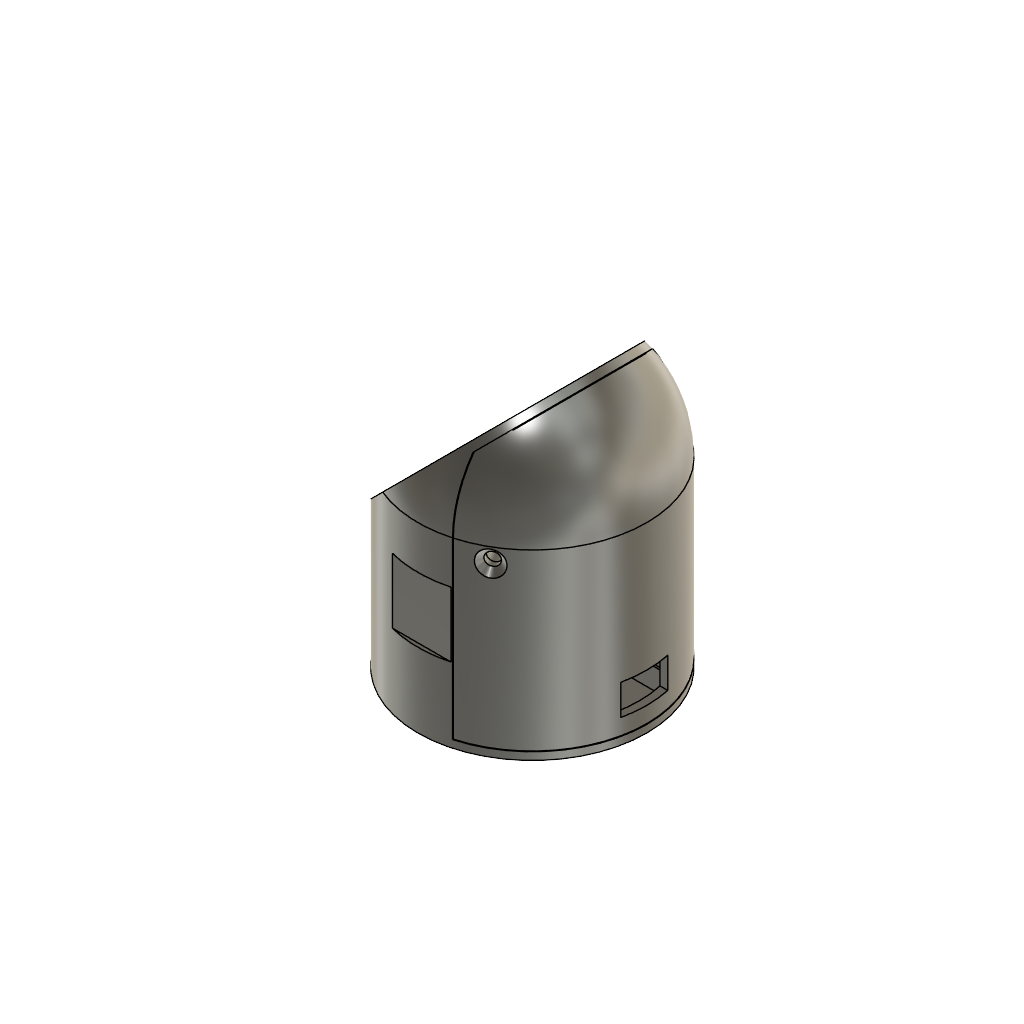
claude_toy (Autodesk Fusion 360 archive; units mm, degrees)
design "claude_bot"
Autodesk Fusion 360 part; units mm, degrees
sketch "Esquisse1" plane through (0, 0, 0) normal (0, 1, 0) x (1, 0, 0)
  line L0 (0, 0) -> (30, 0)
  line L1 (30, 0) -> (30, -47.81)
  arc A0 (0, -77.81) -> (30, -47.81) centre (0, -47.81) ccw
  arc A1 (0, -75.81) -> (28, -47.81) centre (0, -47.81) ccw
  line L2 (28, -2) -> (28, -47.81)
  line L3 (0, -2) -> (28, -2)
  line L4 (0, -77.81) -> (0, -75.81)
  line L5 (0, -2) -> (0, 0)
  line L6 (-0.0898, 1.012) -> (-0.0898, -78.988) construction
  dimension "d3" = 2
  dimension "d17" = 30
  constraint coincident L0.start L5.end
  constraint horizontal L0
  constraint perpendicular L0 L1
  constraint tangent L1 A0
  constraint perpendicular A1 L4
  constraint perpendicular L0 L5
  constraint perpendicular L3 L6
  constraint parallel L4 L6
  constraint coincident L0.start L4
  measures "d17" distance of L0.start L0.end
revolve "Révolution1" add sketch "Esquisse1" angle 360 about axis through (0, 0, 1.75) along (0, 0, 1) makes body 1
ref_plane "Plan de construction4" through (0, 12.125, 0) normal (-0.707107, 0, 0.707107) x (0, 1, 0)
ref_plane "Plan de construction5" through (-28.2843, 12.125, 28.2843) normal (-0.707107, 0, 0.707107) x (0, 1, 0)
split "Scinder1" by plane through (-28.2843, 12.125, 28.2843) normal (-0.707107, 0, 0.707107) bodies 1 makes body 2 at (-10.3059, -28.0164, 50.7878)
sketch "Esquisse3" plane through (-28.2843, 0, 28.2843) normal (-0.707107, 0, 0.707107) x (0, -1, 0)
  ellipse E0 centre (0, 40) end of major axis (0, 82.4264) minor radius 30 (-28.693, 27.6136) -> (28.693, 27.6136) ccw
  arc A0 (28.693, 27.6136) -> (-28.693, 27.6136) centre (0, 33.8068) ccw
  ellipse E1 centre (0, 40) end of major axis (0, 79.598) minor radius 28 (-26.5949, 27.6136) -> (26.5949, 27.6136) ccw
  arc A1 (26.5949, 27.6136) -> (-26.5949, 27.6136) centre (0, 33.8068) ccw
extrude "Extrusion1" add sketch "Esquisse3" along normal blind 2 separate body contours E1 A1 makes body 3
sketch "Esquisse4" plane through (-29.6985, 0, 29.6985) normal (-0.707107, 0, 0.707107) x (0, -1, 0)
  arc A0 (26.5949, 27.6136) -> (-26.5949, 27.6136) centre (0, 33.8068) ccw
  ellipse E0 centre (0, 40) end of major axis (0, 79.598) minor radius 28 (-26.5949, 27.6136) -> (26.5949, 27.6136) ccw
  arc A1 (7.706, 19.3175) -> (-9.294, 19.3175) centre (-0.794, 34.9574) ccw
  line L0 (-9.294, 19.3175) -> (-7.394, 14.6576)
  line L1 (-7.394, 14.6576) -> (-7.394, 14.157)
  line L2 (-7.394, 14.157) -> (5.806, 14.157)
  line L3 (5.806, 14.157) -> (5.806, 14.6576)
  line L4 (5.806, 14.6576) -> (7.706, 19.3175)
  line L5 (-9.4523, 19.176) -> (-7.594, 14.6184)
  line L6 (-7.594, 14.6184) -> (-7.594, 13.957)
  line L7 (-7.594, 13.957) -> (6.006, 13.957)
  line L8 (6.006, 13.957) -> (6.006, 14.6184)
  line L9 (6.006, 14.6184) -> (7.8643, 19.176)
  arc A2 (7.8643, 19.176) -> (-9.4523, 19.176) centre (-0.794, 34.9574) ccw
  dimension "d18" = 0.2
extrude "Decoupe ecran" cut sketch "Esquisse4" against normal blind 3 contours A1 L0 L1 L2 L3 L4 | L5 L6 L7 L8 L9 A2 bodies 3
ref_plane "Plan de construction6" through (0, 26, 0) normal (0, 1, 0) x (0, 0, 1)
sketch "Esquisse8" plane through (0, 26, 0) normal (0, 1, 0) x (1, 0, 0)
  line L0 (-7.5, -18.5) -> (7.5, -18.5)
  line L1 (7.5, -18.5) -> (7.5, -37.5)
  line L2 (7.5, -37.5) -> (-7.5, -37.5)
  line L3 (-7.5, -37.5) -> (-7.5, -18.5)
extrude "Bossage capteur droite" add sketch "Esquisse8" along normal blind 3 bodies 1
ref_plane "Plan de construction7" through (0, 29, 0) normal (0, 1, 0) x (0, 0, 1)
sketch "Esquisse9" plane through (0, 29, 0) normal (0, 1, 0) x (1, 0, 0)
  line L0 (-9, -19.5) -> (9, -19.5)
  line L1 (9, -19.5) -> (9, -36.5)
  line L2 (9, -36.5) -> (-9, -36.5)
  line L3 (-9, -36.5) -> (-9, -19.5)
extrude "Meplat capteur droite" cut sketch "Esquisse9" along normal blind 2 bodies 1
ref_plane "Plan de construction8" through (0, 25.5, 0) normal (0, 1, 0) x (0, 0, 1)
sketch "Esquisse10" plane through (0, 25.5, 0) normal (0, 1, 0) x (1, 0, 0)
  line L0 (-5.53, -20.6) -> (5.53, -20.6)
  line L1 (5.53, -20.6) -> (5.53, -35.4)
  line L2 (5.53, -35.4) -> (-5.53, -35.4)
  line L3 (-5.53, -35.4) -> (-5.53, -20.6)
extrude "Logement capteur droite" cut sketch "Esquisse10" along normal blind 3 bodies 1
ref_plane "Plan de construction9" through (0, -26, 0) normal (0, 1, 0) x (0, 0, 1)
sketch "Esquisse11" plane through (0, -26, 0) normal (0, 1, 0) x (1, 0, 0)
  line L0 (-7.5, -18.5) -> (7.5, -18.5)
  line L1 (7.5, -18.5) -> (7.5, -37.5)
  line L2 (7.5, -37.5) -> (-7.5, -37.5)
  line L3 (-7.5, -37.5) -> (-7.5, -18.5)
extrude "Bossage capteur gauche" add sketch "Esquisse11" against normal blind 3 bodies 1
ref_plane "Plan de construction10" through (0, -29, 0) normal (0, 1, 0) x (0, 0, 1)
sketch "Esquisse12" plane through (0, -29, 0) normal (0, 1, 0) x (1, 0, 0)
  line L0 (-9, -19.5) -> (9, -19.5)
  line L1 (9, -19.5) -> (9, -36.5)
  line L2 (9, -36.5) -> (-9, -36.5)
  line L3 (-9, -36.5) -> (-9, -19.5)
extrude "Meplat capteur gauche" cut sketch "Esquisse12" against normal blind 2 bodies 1
ref_plane "Plan de construction11" through (0, -25.5, 0) normal (0, 1, 0) x (0, 0, 1)
sketch "Esquisse13" plane through (0, -25.5, 0) normal (0, 1, 0) x (1, 0, 0)
  line L0 (-5.53, -20.6) -> (5.53, -20.6)
  line L1 (5.53, -20.6) -> (5.53, -35.4)
  line L2 (5.53, -35.4) -> (-5.53, -35.4)
  line L3 (-5.53, -35.4) -> (-5.53, -20.6)
extrude "Logement capteur gauche" cut sketch "Esquisse13" against normal blind 3 bodies 1
ref_plane "Plan de construction12" through (0, 0, 1) normal (0, 0, 1) x (1, 0, 0)
sketch "Esquisse14" plane through (0, 0, 1) normal (0, 0, 1) x (1, 0, 0)
  line L0 (2.55, 9.15) -> (25.4, 9.15)
  line L1 (25.4, 9.15) -> (25.4, 10.65)
  line L2 (25.4, 10.65) -> (2.55, 10.65)
  line L3 (2.55, 10.65) -> (2.55, 9.15)
  line L4 (2.55, -10.65) -> (25.4, -10.65)
  line L5 (25.4, -10.65) -> (25.4, -9.15)
  line L6 (25.4, -9.15) -> (2.55, -9.15)
  line L7 (2.55, -9.15) -> (2.55, -10.65)
  line L8 (1.05, -10.65) -> (2.55, -10.65)
  line L9 (2.55, -10.65) -> (2.55, 10.65)
  line L10 (2.55, 10.65) -> (1.05, 10.65)
  line L11 (1.05, 10.65) -> (1.05, -10.65)
extrude "Berceau ESP parois" add sketch "Esquisse14" along normal blind 9.1 bodies 1
ref_plane "Plan de construction13" through (0, 0, 1) normal (0, 0, 1) x (1, 0, 0)
sketch "Esquisse15" plane through (0, 0, 1) normal (0, 0, 1) x (1, 0, 0)
  line L0 (2.7, 8.6) -> (25.4, 8.6)
  line L1 (25.4, 8.6) -> (25.4, 9.15)
  line L2 (25.4, 9.15) -> (2.7, 9.15)
  line L3 (2.7, 9.15) -> (2.7, 8.6)
  line L4 (2.7, -9.15) -> (25.4, -9.15)
  line L5 (25.4, -9.15) -> (25.4, -8.6)
  line L6 (25.4, -8.6) -> (2.7, -8.6)
  line L7 (2.7, -8.6) -> (2.7, -9.15)
extrude "Berceau ESP appuis" add sketch "Esquisse15" along normal blind 6.5 bodies 1
ref_plane "Plan de construction14" through (0, 0, 9.21) normal (0, 0, 1) x (1, 0, 0)
sketch "Esquisse16" plane through (0, 0, 9.21) normal (0, 0, 1) x (1, 0, 0)
  line L0 (12.45, 8.6) -> (16.45, 8.6)
  line L1 (16.45, 8.6) -> (16.45, 9.15)
  line L2 (16.45, 9.15) -> (12.45, 9.15)
  line L3 (12.45, 9.15) -> (12.45, 8.6)
  line L4 (12.45, -9.15) -> (16.45, -9.15)
  line L5 (16.45, -9.15) -> (16.45, -8.6)
  line L6 (16.45, -8.6) -> (12.45, -8.6)
  line L7 (12.45, -8.6) -> (12.45, -9.15)
extrude "Clips ESP" add sketch "Esquisse16" along normal blind 0.4 bodies 1
ref_plane "Plan de construction15" through (27, 0, 0) normal (1, 0, 0) x (0, 1, 0)
sketch "Esquisse18" plane through (0, 0, 9.21) normal (0, 0, 1) x (1, 0, 0)
  line L0 (12.45, 8.6) -> (16.45, 8.6)
  line L1 (16.45, 8.6) -> (16.45, 8.85)
  line L2 (16.45, 8.85) -> (12.45, 8.85)
  line L3 (12.45, 8.85) -> (12.45, 8.6)
  line L4 (12.45, -8.85) -> (16.45, -8.85)
  line L5 (16.45, -8.85) -> (16.45, -8.6)
  line L6 (16.45, -8.6) -> (12.45, -8.6)
  line L7 (12.45, -8.6) -> (12.45, -8.85)
extrude "Clips ESP extension" add sketch "Esquisse18" along normal blind 0.4 bodies 1
sketch "Esquisse19" plane through (27, 0, 0) normal (1, 0, 0) x (0, 0, -1)
  line L0 (-6.31, -6.15) -> (-14.31, -6.15)
  line L1 (-14.31, -6.15) -> (-14.31, 6.15)
  line L2 (-14.31, 6.15) -> (-6.31, 6.15)
  line L3 (-6.31, 6.15) -> (-6.31, -6.15)
extrude "Passage USB-C" cut sketch "Esquisse19" along normal blind 4 bodies 1
ref_plane "Plan de construction16" through (0, 28.5, 0) normal (0, 1, 0) x (0, 0, 1)
ref_plane "Plan de construction17" through (0, -28.5, 0) normal (0, 1, 0) x (0, 0, 1)
ref_plane "Plan de construction18" through (0, 0, 2) normal (0, 0, 1) x (1, 0, 0)
ref_plane "Plan de construction19" through (0, 0, 2.15) normal (0, 0, 1) x (1, 0, 0)
sketch "Esquisse22" plane through (0, 0, 2) normal (0, 0, 1) x (1, 0, 0)
  line L0 (8, -31) -> (31, -31)
  line L1 (31, -31) -> (31, 31)
  line L2 (31, 31) -> (8, 31)
  line L3 (8, 31) -> (8, -31)
extrude "Outil coupe principal" add sketch "Esquisse22" along normal blind 78 separate body makes body 4
sketch "Esquisse23" plane through (0, 0, 2) normal (0, 0, 1) x (1, 0, 0)
  line L0 (8, -11) -> (25.5, -11)
  line L1 (25.5, -11) -> (25.5, 11)
  line L2 (25.5, 11) -> (8, 11)
  line L3 (8, 11) -> (8, -11)
extrude "Outil reserve berceau" cut sketch "Esquisse23" along normal blind 9 bodies 4
sketch "Esquisse24" plane through (0, 0, 2.15) normal (0, 0, 1) x (1, 0, 0)
  line L0 (8.15, -31) -> (31, -31)
  line L1 (31, -31) -> (31, 31)
  line L2 (31, 31) -> (8.15, 31)
  line L3 (8.15, 31) -> (8.15, -31)
extrude "Outil coupe trappe" add sketch "Esquisse24" along normal blind 77.85 separate body makes body 5
sketch "Esquisse25" plane through (0, 0, 2.15) normal (0, 0, 1) x (1, 0, 0)
  line L0 (8, -11.15) -> (25.65, -11.15)
  line L1 (25.65, -11.15) -> (25.65, 11.15)
  line L2 (25.65, 11.15) -> (8, 11.15)
  line L3 (8, 11.15) -> (8, -11.15)
extrude "Outil reserve berceau jeu" cut sketch "Esquisse25" along normal blind 9 bodies 5
sketch "Esquisse26" plane through (0, 0, 0) normal (0, 1, 0) x (1, 0, 0)
  line L0 (5, -61.3564) -> (40, -96.3564)
  line L1 (40, -96.3564) -> (5, -96.3564)
  line L2 (5, -96.3564) -> (5, -61.3564)
extrude "Outil jeu facade" cut sketch "Esquisse26" along normal mid plane 35 bodies 5
sketch "Esquisse37" plane through (0, 0, 0) normal (0, 1, 0) x (1, 0, 0)
  line L0 (28, -2) -> (29, -2)
  line L1 (29, -2) -> (29, -47.81)
  arc A0 (0, -76.81) -> (29, -47.81) centre (0, -47.81) ccw
  line L2 (0, -76.81) -> (0, -75.81)
  arc A1 (0, -75.81) -> (28, -47.81) centre (0, -47.81) ccw
  line L3 (28, -47.81) -> (28, -2)
revolve "Outil levre principal" add sketch "Esquisse37" angle 360 about axis through (0, 0, 1.75) along (0, 0, 1) separate body makes body 6
ref_plane "Plan de construction25" through (0, 0, 1) normal (0, 0, 1) x (1, 0, 0)
sketch "Esquisse38" plane through (0, 0, 1) normal (0, 0, 1) x (1, 0, 0)
  line L0 (8, -32) -> (11, -32)
  line L1 (11, -32) -> (11, 32)
  line L2 (11, 32) -> (8, 32)
  line L3 (8, 32) -> (8, -32)
extrude "Boite levre principal" add sketch "Esquisse38" along normal blind 80 separate body makes body 7
combine "Levre principal limite" operation intersect target body 6 tool bodies 7
sketch "Esquisse39" plane through (0, 0, 0) normal (0, 1, 0) x (1, 0, 0)
  line L0 (27.85, -1.9) -> (29.15, -1.9)
  line L1 (29.15, -1.9) -> (29.15, -47.81)
  arc A0 (0, -76.96) -> (29.15, -47.81) centre (0, -47.81) ccw
  line L2 (0, -76.96) -> (0, -75.66)
  arc A1 (0, -75.66) -> (27.85, -47.81) centre (0, -47.81) ccw
  line L3 (27.85, -47.81) -> (27.85, -1.9)
revolve "Outil levre trappe" add sketch "Esquisse39" angle 360 about axis through (0, 0, 1.75) along (0, 0, 1) separate body makes body 8
ref_plane "Plan de construction26" through (0, 0, 1) normal (0, 0, 1) x (1, 0, 0)
sketch "Esquisse40" plane through (0, 0, 1) normal (0, 0, 1) x (1, 0, 0)
  line L0 (7, -32) -> (11.15, -32)
  line L1 (11.15, -32) -> (11.15, 32)
  line L2 (11.15, 32) -> (7, 32)
  line L3 (7, 32) -> (7, -32)
extrude "Boite levre trappe" add sketch "Esquisse40" along normal blind 80 separate body makes body 9
combine "Levre trappe limite" operation intersect target body 8 tool bodies 9
combine "Outil principal moins levre" operation cut target body 4 tool bodies 6
combine "Outil trappe moins rainure" operation cut target body 5 tool bodies 8
copy_body "CopierCollerCorps1" bodies 1 makes body 10
combine "Creation trappe" operation intersect target body 10 tool bodies 5
combine "Separation trappe" operation cut target body 1 tool bodies 4
ref_plane "Plan de construction20" through (0, 0, 39) normal (0, 0, 1) x (1, 0, 0)
ref_plane "Plan de construction21" through (0, 0, 40) normal (0, 0, 1) x (1, 0, 0)
sketch "Esquisse27" plane through (0, 0, 39) normal (0, 0, 1) x (1, 0, 0)
  arc A0 (13.6271, 16.2401) -> (1.8477, 21.1193) centre (0, 0) ccw
  arc A1 (17.1624, 20.4534) -> (2.3271, 26.5984) centre (0, 0) ccw
  line L0 (13.6271, 16.2401) -> (17.1624, 20.4534)
  line L1 (1.8477, 21.1193) -> (2.3271, 26.5984)
extrude "Patte vis gauche" add sketch "Esquisse27" along normal blind 10 bodies 1 makes body 11
sketch "Esquisse28" plane through (0, 0, 39) normal (0, 0, 1) x (1, 0, 0)
  arc A0 (6.8587, 25.597) -> (2.3096, 26.3992) centre (0, 0) ccw
  arc A1 (7.6352, 28.4948) -> (2.5711, 29.3877) centre (0, 0) ccw
  line L0 (6.8587, 25.597) -> (7.6352, 28.4948)
  line L1 (2.3096, 26.3992) -> (2.5711, 29.3877)
extrude "Attache patte gauche" add sketch "Esquisse28" along normal blind 10 bodies 1
sketch "Esquisse30" plane through (0, 0, 39) normal (0, 0, 1) x (1, 0, 0)
  arc A0 (1.8477, -21.1193) -> (13.6271, -16.2401) centre (0, 0) ccw
  arc A1 (2.3271, -26.5984) -> (17.1624, -20.4534) centre (0, 0) ccw
  line L0 (13.6271, -16.2401) -> (17.1624, -20.4534)
  line L1 (1.8477, -21.1193) -> (2.3271, -26.5984)
extrude "Patte vis droite" add sketch "Esquisse30" along normal blind 10 bodies 1 makes body 12
sketch "Esquisse31" plane through (0, 0, 39) normal (0, 0, 1) x (1, 0, 0)
  arc A0 (2.3096, -26.3992) -> (6.8587, -25.597) centre (0, 0) ccw
  arc A1 (2.5711, -29.3877) -> (7.6352, -28.4948) centre (0, 0) ccw
  line L0 (6.8587, -25.597) -> (7.6352, -28.4948)
  line L1 (2.3096, -26.3992) -> (2.5711, -29.3877)
extrude "Attache patte droite" add sketch "Esquisse31" along normal blind 10 bodies 1
combine "Fusion pattes vis" operation add target body 1 tool bodies 11 12
sketch "Esquisse41" plane through (0, 0, 40) normal (0, 0, 1) x (1, 0, 0)
  arc A0 (16.1587, 21.4434) -> (11.3473, 24.3344) centre (0, 0) ccw
  arc A1 (17.6332, 23.4) -> (12.3827, 26.5548) centre (0, 0) ccw
  line L0 (16.1587, 21.4434) -> (17.6332, 23.4)
  line L1 (11.3473, 24.3344) -> (12.3827, 26.5548)
extrude "Bossage vis trappe gauche" add sketch "Esquisse41" along normal blind 8 bodies 10
sketch "Esquisse42" plane through (0, 0, 40) normal (0, 0, 1) x (1, 0, 0)
  arc A0 (11.3473, -24.3344) -> (16.1587, -21.4434) centre (0, 0) ccw
  arc A1 (12.3827, -26.5548) -> (17.6332, -23.4) centre (0, 0) ccw
  line L0 (16.1587, -21.4434) -> (17.6332, -23.4)
  line L1 (11.3473, -24.3344) -> (12.3827, -26.5548)
extrude "Bossage vis trappe droite" add sketch "Esquisse42" along normal blind 8 bodies 10
ref_plane "Plan de construction22" through (0, 0, 12.125) normal (-0.866025, 0.5, 0) x (0, 0, 1)
sketch "Esquisse33" plane through (0, 0, 0) normal (-0.866025, 0.5, 0) x (0, 0, 1)
  line L0 (44, 15) -> (44, 33) construction
  line L1 (44, 26.4) -> (45.7, 26.4)
  line L2 (45.7, 26.4) -> (45.7, 28.4)
  line L3 (45.7, 28.4) -> (47.3, 30)
  line L4 (47.3, 30) -> (47.3, 31.5)
  line L5 (47.3, 31.5) -> (44, 31.5)
  line L6 (44, 31.5) -> (44, 26.4)
revolve "Percage fraise trappe gauche" cut sketch "Esquisse33" angle 360 about axis through (7.5, 12.9904, 44) along (0.5, 0.866025, 0) bodies 10
sketch "Esquisse34" plane through (0, 0, 0) normal (-0.866025, 0.5, 0) x (0, 0, 1)
  line L0 (44, 15) -> (44, 33) construction
  line L1 (44, 27) -> (46, 27)
  line L2 (46, 27) -> (46, 22.2)
  line L3 (46, 22.2) -> (45.4, 22.2)
  line L4 (45.4, 22.2) -> (45.4, 20.5)
  line L5 (45.4, 20.5) -> (44, 20.5)
  line L6 (44, 20.5) -> (44, 27)
revolve "Logement insert gauche" cut sketch "Esquisse34" angle 360 about axis through (7.5, 12.9904, 44) along (0.5, 0.866025, 0) bodies 1
ref_plane "Plan de construction24" through (0, 0, 12.125) normal (0.866025, 0.5, 0) x (0, 0, 1)
sketch "Esquisse35" plane through (0, 0, 0) normal (0.866025, 0.5, 0) x (0, 0, 1)
  line L0 (44, 15) -> (44, 33) construction
  line L1 (44, 26.4) -> (45.7, 26.4)
  line L2 (45.7, 26.4) -> (45.7, 28.4)
  line L3 (45.7, 28.4) -> (47.3, 30)
  line L4 (47.3, 30) -> (47.3, 31.5)
  line L5 (47.3, 31.5) -> (44, 31.5)
  line L6 (44, 31.5) -> (44, 26.4)
revolve "Percage fraise trappe droite" cut sketch "Esquisse35" angle 360 about axis through (7.5, -12.9904, 44) along (0.5, -0.866025, 0) bodies 10
sketch "Esquisse36" plane through (0, 0, 0) normal (0.866025, 0.5, 0) x (0, 0, 1)
  line L0 (44, 15) -> (44, 33) construction
  line L1 (44, 27) -> (46, 27)
  line L2 (46, 27) -> (46, 22.2)
  line L3 (46, 22.2) -> (45.4, 22.2)
  line L4 (45.4, 22.2) -> (45.4, 20.5)
  line L5 (45.4, 20.5) -> (44, 20.5)
  line L6 (44, 20.5) -> (44, 27)
revolve "Logement insert droite" cut sketch "Esquisse36" angle 360 about axis through (7.5, -12.9904, 44) along (0.5, -0.866025, 0) bodies 1
combine "Fusion corps + facade" operation add target body 1 tool bodies 3
split "Decoupe anneau facade" by plane through (-29.6985, 0, 29.6985) normal (-0.707107, 0, 0.707107) bodies 2 makes body 13 at (-29.7433, 0, 51.7258)
delete_body "RemoveBody2" bodies 13
combine "Fusion anneau facade" operation add target body 1 tool bodies 2
ref_plane "Plan de construction27" through (-28.2843, 12.125, 28.2843) normal (-0.707107, 0, 0.707107) x (0, 1, 0)
sketch "Esquisse43" plane through (-28.2843, 0, 28.2843) normal (-0.707107, 0, 0.707107) x (0, 1, 0)
  line L0 (-10.936, -9.422) -> (-10.936, -19.2327)
  arc A0 (-10.936, -19.2327) -> (12.524, -19.2327) centre (0.794, -34.622) ccw
  line L1 (12.524, -19.2327) -> (12.524, -9.422)
  arc A1 (12.524, -9.422) -> (10.974, -7.872) centre (10.974, -9.422) ccw
  line L2 (10.974, -7.872) -> (-9.386, -7.872)
  arc A2 (-9.386, -7.872) -> (-10.936, -9.422) centre (-9.386, -9.422) ccw
extrude "Lamage ecran" cut sketch "Esquisse43" along normal blind 0.9 bodies 1
ref_plane "Plan de construction28" through (-28.9207, 12.125, 28.9207) normal (-0.707107, 0, 0.707107) x (0, 1, 0)
sketch "Esquisse44" plane through (-28.9207, 0, 28.9207) normal (-0.707107, 0, 0.707107) x (0, 1, 0)
  circle A0 centre (-8.636, -12.952) radius 2.25
  circle A1 centre (-8.636, -12.952) radius 0.9
  circle A2 centre (10.224, -12.952) radius 2.25
  circle A3 centre (10.224, -12.952) radius 0.9
extrude "Epaulements plots" add sketch "Esquisse44" against normal blind 0.5 contours A0 | A1 | A2 | A3 bodies 1
extrude "Pions scellage" add sketch "Esquisse44" against normal blind 3.6 contours A1 | A3 bodies 1
sketch "Esquisse45" plane through (-28.9207, 0, 28.9207) normal (-0.707107, 0, 0.707107) x (0, 1, 0)
  line L0 (-8, -7.95) -> (9.6, -7.95)
  line L1 (9.6, -7.95) -> (9.6, -11.15)
  line L2 (9.6, -11.15) -> (-8, -11.15)
  line L3 (-8, -11.15) -> (-8, -7.95)
  line L4 (-5.21, -12.5) -> (6.79, -12.5)
  line L5 (6.79, -12.5) -> (6.79, -14.3)
  line L6 (6.79, -14.3) -> (-5.21, -14.3)
  line L7 (-5.21, -14.3) -> (-5.21, -12.5)
extrude "Poches connecteur et nappe" cut sketch "Esquisse45" along normal blind 0.4 bodies 1
sketch "Esquisse46" plane through (-28.9207, 0, 28.9207) normal (-0.707107, 0, 0.707107) x (0, 1, 0)
  line L0 (-5.21, -13.5) -> (6.79, -13.5)
  line L1 (6.79, -13.5) -> (6.79, -14.1)
  line L2 (6.79, -14.1) -> (-5.21, -14.1)
  line L3 (-5.21, -14.1) -> (-5.21, -13.5)
extrude "Passage nappe" cut sketch "Esquisse46" along normal blind 1.5 bodies 1
equation "d19 = -( 3 mm )"
equation "d43 = -( 3.000 mm )"
equation "d47 = -( 2.000 mm )"
equation "d51 = -( 3.000 mm )"
equation "d141 = -( 0.500 mm )"
equation "d143 = -( 3.600 mm )"
named bodies: "Corps principal", "Anneau facade", "Outil principal", "Outil trappe", "Trappe"
